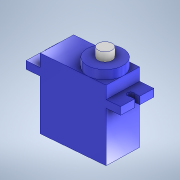
# Autodesk Inventor part: FS90R
Saved by Autodesk Inventor 2022 (Build 260153000, 153)
## iProperties
Created: 2024-05-30
Part Number: FS90R
Material: 一般
Document SubType Name: Modeling
Designer: yamashita1
Density: 1 g/cm^3
Appearance: 青 - 壁塗料 - 光沢
HEIGHT: 12.100 mm
WIDTH: 22.500 mm
DEPTH: 23.400 mm
TAB_DEPTH: -16.700 mm
TAB_THIN: 2.500 mm
Author: yamashita1
Autodesk Inventor part; units mm, degrees
ref_plane "YZ Plane" through (0, 0, 0) normal (1, 0, 0) x (0, 1, 0)
ref_plane "XZ Plane" through (0, 0, 0) normal (0, 1, 0) x (-1, 0, 0)
sketch "スケッチ1" plane through (0, 0, 0) normal (0, 0, 1) x (1, 0, 0)
  line L0 (-19, 8.4016) -> (-19, -8.0875) construction
  line L1 (0, -8.2446) -> (0, 8.2446) construction
  line L2 (8.7, 8.4016) -> (8.7, -8.0875) construction
  circle A0 centre (0, 0) radius 6.05
  line L3 (6.05, 6.05) -> (-16.45, 6.05)
  line L4 (-16.45, 6.05) -> (-16.45, -6.05)
  line L5 (-16.45, -6.05) -> (6.05, -6.05)
  line L6 (6.05, -6.05) -> (6.05, 6.05)
  point P0 (6.05, 0)
  dimension "HEIGHT" = 12.1
  dimension "d0" = 8.7
  dimension "d1" = 27.7
  dimension "WIDTH" = 22.5
  constraints: 14 end point, 3 horizontal, 2 coincident, 2 midpoint, 2 parallel, 1 horizontal alignment, 1 perpendicular, 1 vertical, 2 other
  measures "d0" distance between parallel lines of L2 L1
  measures "d1" distance between parallel lines of L0 L2
  measures "WIDTH" distance of L3.start L3.end
extrude "軸台" add sketch "スケッチ1" along normal blind 3 contours A0
extrude "本体" add sketch "スケッチ1" against normal blind 23.4
ref_plane "作業平面1" through (0, 0, -6.7) normal (0, 0, -1) x (-1, 0, 0)
sketch "スケッチ2" plane through (0, 0, -6.7) normal (0, 0, -1) x (-1, 0, 0)
  line L0 (-11, 6.05) -> (21.3, 6.05)
  line L1 (21.3, 6.05) -> (21.3, -6.05)
  line L2 (21.3, -6.05) -> (-11, -6.05)
  line L3 (-11, -6.05) -> (-11, 6.05)
  line L4 (-6.05, 6.05) -> (0, 6.05) projected
  line L5 (0, -6.05) -> (-6.05, -6.05) projected
  circle A0 centre (19, 0) radius 1.1
  circle A1 centre (-8.7, 0) radius 1.1
  line L6 (-8.7, 8.0806) -> (-8.7, -7.6301) construction
  line L7 (19, -7.6301) -> (19, 8.0806) construction
  line L8 (5.15, 8.0806) -> (5.15, -7.8882) construction
  line L9 (-11, 0.9) -> (-9.3325, 0.9)
  line L10 (-9.3325, 0.9) -> (-9.3325, -0.9)
  line L11 (-9.3325, -0.9) -> (-11, -0.9)
  line L12 (-11, -0.9) -> (-11, 0.9)
  line L13 (19.6325, 0.9) -> (21.3, 0.9)
  line L14 (21.3, 0.9) -> (21.3, -0.9)
  line L15 (21.3, -0.9) -> (19.6325, -0.9)
  line L16 (19.6325, -0.9) -> (19.6325, 0.9)
  point P0 (0, 0)
  point P1 (5.15, 6.05)
  point P2 (-11, 0)
  point P3 (21.3, 0)
  dimension "d10" = 2.2
  dimension "d9" = 32.3
  dimension "d11" = 8.7
  dimension "d12" = 27.7
  dimension "d13" = 1.8
  constraints: 30 end point, 7 parallel, 5 midpoint, 3 horizontal, 3 perpendicular, 3 point on line, 2 collinear, 2 horizontal alignment, 2 vertical, 7 other
  measures "d9" distance of L0.start L0.end
  measures "d11" distance from line of point (0, 0) L6
  measures "d12" distance between parallel lines of L7 L6
  measures "d13" distance of L9.end L10.end
extrude "タブ" add sketch "スケッチ2" against normal blind 2.5 contours L0 L1 L13 A0 L15 L2 L3 L11 A1 L9
sketch "スケッチ3" plane through (0, 0, 3) normal (0, 0, 1) x (1, 0, 0)
  circle A0 centre (0, 0) radius 2.43
  dimension "d16" = 4.86
  constraints: 1 centre point, 1 coincident
  measures "d16" diameter of A0
extrude "軸" add sketch "スケッチ3" along normal blind 3
equation "\"d11\" = d0"
equation "\"d12\" = d1"
